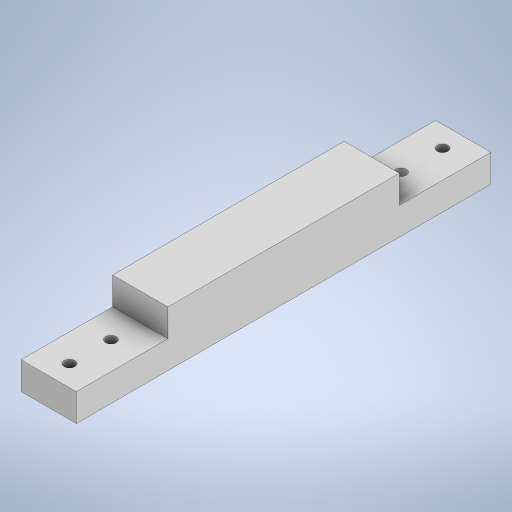
# Autodesk Inventor part: A_base
Saved by Autodesk Inventor 2023.1 (Build 271208000, 208)
## iProperties
Created: 2023-06-14
Part Number: A_base
Material: Generic
Document SubType Name: Modeling
Designer: zavrel
Density: 1 g/cm^3
Appearance: Default
Author: zavrel
Autodesk Inventor part; units mm, degrees
ref_plane "YZ Plane" through (0, 0, 0) normal (1, 0, 0) x (0, 1, 0)
ref_plane "XZ Plane" through (0, 0, 0) normal (0, 1, 0) x (-1, 0, 0)
ref_plane "XY Plane" through (0, 0, 0) normal (0, 0, 1) x (1, 0, 0)
sketch "Sketch1" plane through (0, 0, 0) normal (0, 1, 0) x (-1, 0, 0)
  line L0 (0, 0) -> (16, 0)
  line L1 (16, 0) -> (16, -120)
  line L2 (16, -120) -> (0, -120)
  line L3 (0, -120) -> (0, 0)
  dimension "d0" = 120
  dimension "d1" = 16
  constraints: 8 end point, 2 parallel, 1 horizontal, 1 perpendicular
  measures "d0" distance of L0.end L1.end
  measures "d1" distance of L1.end L2.end
extrude "Extrusion" add sketch "Sketch1" along normal blind 16
sketch "Sketch2" plane through (0, 16, 0) normal (0, 1, 0) x (1, 0, 0)
  line L0 (0, 120) -> (-16, 120) projected
  line L1 (-16, 120) -> (-16, 0) projected
  line L2 (-16, 0) -> (0, 0) projected
  line L3 (0, 0) -> (0, 120) projected
  line L4 (-16, 120) -> (-16, 0) projected
  line L5 (-16, 0) -> (0, 0)
  line L6 (0, 0) -> (0, 26.5)
  line L7 (0, 26.5) -> (-16, 26.5)
  line L8 (-16, 26.5) -> (-16, 0)
  line L9 (0, 0) -> (0, 120) projected
  line L10 (-16, 120) -> (0, 120)
  line L11 (0, 120) -> (0, 93.5)
  line L12 (0, 93.5) -> (-16, 93.5)
  line L13 (-16, 93.5) -> (-16, 120)
  point P0 (-8, 26.5)
  point P1 (-16, 93.5)
  point P2 (-16, 26.5)
  dimension "d4" = 26.5
  dimension "d5" = 26.5
  constraints: 16 end point, 4 parallel, 2 horizontal, 2 perpendicular, 2 point on line, 1 midpoint
  measures "d4" distance from line of L2 point (-8, 26.5)
  measures "d5" distance between parallel lines of L0 L12
extrude "Extrusion2" cut sketch "Sketch2" against normal blind 8 contours L3 L12 L1 L0 | L3 L2 L1 L7
sketch "Sketch3" plane through (0, 0, 0) normal (0, -1, 0) x (1, 0, 0)
  line L0 (0, -120) -> (-16, -120) projected
  line L1 (0, 0) -> (0, -120) projected
  line L2 (-16, 0) -> (0, 0) projected
  line L3 (-16, -120) -> (-16, 0) projected
  circle A0 centre (-8, -6) radius 1.55
  line L4 (0, -26.5) -> (0, -93.5) construction
  line L5 (0, -60) -> (-16, -60) construction
  line L6 (-16, -120) -> (-16, 0) construction
  circle A1 centre (-8, -18) radius 1.55
  circle A2 centre (-8, -114) radius 1.55
  circle A3 centre (-8, -102) radius 1.55
  dimension "d8" = 3.1
  dimension "d9" = 8
  dimension "d10" = 6
  dimension "d11" = 12
  constraints: 4 centre point, 2 end point, 2 midpoint, 2 symmetric about line, 1 equal radius, 2 other
  measures "d8" diameter of A0
  measures "d9" distance from line of L1 A0.centre
  measures "d10" distance from line of L2 A0.centre
  measures "d11" distance of A1.centre A0.centre
extrude "Extrusion3" cut sketch "Sketch3" against normal through all contours A0 | A1 | A2 | A3
sketch "Sketch4" plane through (0, 0, 0) normal (0, -1, 0) x (1, 0, 0)
  circle A0 centre (-8, -6) radius 1.55 projected
  circle A1 centre (-8, -114) radius 1.55 projected
  circle A2 centre (-8, -18) radius 1.55 projected
  circle A3 centre (-8, -102) radius 1.55 projected
  line L0 (0, -120) -> (-16, -120) projected
  line L1 (0, 0) -> (0, -120) projected
  line L2 (-16, 0) -> (0, 0) projected
  line L3 (-16, -120) -> (-16, 0) projected
  circle A4 centre (-8, -6) radius 1.55 projected
  line L4 (-8, -2.7668) -> (-5.2, -4.3834)
  line L5 (-5.2, -4.3834) -> (-5.2, -7.6166)
  line L6 (-5.2, -7.6166) -> (-8, -9.2332)
  line L7 (-8, -9.2332) -> (-10.8, -7.6166)
  line L8 (-10.8, -7.6166) -> (-10.8, -4.3834)
  line L9 (-10.8, -4.3834) -> (-8, -2.7668)
  line L10 (-8, -14.7668) -> (-5.2, -16.3834)
  line L11 (-5.2, -16.3834) -> (-5.2, -19.6166)
  line L12 (-5.2, -19.6166) -> (-8, -21.2332)
  line L13 (-8, -21.2332) -> (-10.8, -19.6166)
  line L14 (-10.8, -19.6166) -> (-10.8, -16.3834)
  line L15 (-10.8, -16.3834) -> (-8, -14.7668)
  line L16 (-8, -98.7668) -> (-5.2, -100.3834)
  line L17 (-5.2, -100.3834) -> (-5.2, -103.6166)
  line L18 (-5.2, -103.6166) -> (-8, -105.2332)
  line L19 (-8, -105.2332) -> (-10.8, -103.6166)
  line L20 (-10.8, -103.6166) -> (-10.8, -100.3834)
  line L21 (-10.8, -100.3834) -> (-8, -98.7668)
  line L22 (-8, -110.7668) -> (-5.2, -112.3834)
  line L23 (-5.2, -112.3834) -> (-5.2, -115.6166)
  line L24 (-5.2, -115.6166) -> (-8, -117.2332)
  line L25 (-8, -117.2332) -> (-10.8, -115.6166)
  line L26 (-10.8, -115.6166) -> (-10.8, -112.3834)
  line L27 (-10.8, -112.3834) -> (-8, -110.7668)
  dimension "d14" = 5.6
  dimension "d15" = 5.6
  dimension "d16" = 5.6
  dimension "d17" = 5.6
  constraints: 48 end point, 1 coincident, 13 other
  measures "d14" distance between parallel lines of L8 L5
  measures "d15" distance between parallel lines of L14 L11
  measures "d16" distance between parallel lines of L20 L17
  measures "d17" distance between parallel lines of L26 L23
extrude "Extrusion4" cut sketch "Sketch4" against normal blind 2.5 contours L4 L5 L6 L7 L8 L9 | L10 L11 L12 L13 L14 L15 | L16 L17 L18 L19 L20 L21 | L22 L23 L24 L25 L26 L27
body "Solid1"
